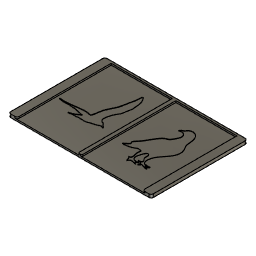
Wingspan - Lid alt (Autodesk Fusion 360 design; units mm, degrees)
Autodesk Fusion 360 part; units mm, degrees
sketch "Skizze1" plane through (0, 0, 0) normal (0, 0, 1) x (1, 0, 0)
  line L0 (0, 0) -> (135.5, 0)
  line L1 (135.5, 0) -> (135.5, 91.5)
  line L2 (135.5, 91.5) -> (0, 91.5)
  line L3 (0, 91.5) -> (0, 0)
  line L4 (0, 0) -> (7, 0)
  line L5 (7, 0) -> (7, 7)
  line L6 (7, 7) -> (0, 7)
  line L7 (0, 7) -> (0, 0)
  line L8 (135.5, 0) -> (128.5, 0)
  line L9 (128.5, 0) -> (128.5, 7)
  line L10 (128.5, 7) -> (135.5, 7)
  line L11 (135.5, 7) -> (135.5, 0)
  line L12 (135.5, 91.5) -> (128.5, 91.5)
  line L13 (128.5, 91.5) -> (128.5, 84.5)
  line L14 (128.5, 84.5) -> (135.5, 84.5)
  line L15 (135.5, 84.5) -> (135.5, 91.5)
  line L16 (0, 91.5) -> (7, 91.5)
  line L17 (7, 91.5) -> (7, 84.5)
  line L18 (7, 84.5) -> (0, 84.5)
  line L19 (0, 84.5) -> (0, 91.5)
  circle A0 centre (3.5, 88) radius 2.65
  circle A1 centre (132, 88) radius 2.65
  circle A2 centre (132, 3.5) radius 2.65
  circle A3 centre (3.5, 3.5) radius 2.65
  dimension "d1" = 135.5
  dimension "d2" = 91.5
  dimension "d3" = 7
  dimension "d4" = 7
  dimension "d5" = 7
  dimension "d6" = 7
  dimension "d7" = 7
  dimension "d8" = 7
  dimension "d9" = 7
  dimension "d10" = 7
  dimension "d11" = 5.3
  dimension "d12" = 5.3
  dimension "d13" = 5.3
  dimension "d14" = 5.3
  dimension "d15" = 3.5
  dimension "d16" = 3.5
  dimension "d17" = 3.5
  dimension "d18" = 3.5
  dimension "d19" = 3.5
  dimension "d20" = 3.5
  dimension "d21" = 3.5
  dimension "d22" = 3.5
  constraint horizontal L0
  constraint vertical L1
  constraint horizontal L2
  constraint vertical L3
  constraint coincident L0.start L3.end
  constraint horizontal L4
  constraint vertical L5
  constraint horizontal L6
  constraint vertical L7
  constraint horizontal L8
  constraint vertical L9
  constraint horizontal L10
  constraint vertical L11
  constraint horizontal L12
  constraint vertical L13
  constraint horizontal L14
  constraint vertical L15
  constraint horizontal L16
  constraint vertical L17
  constraint horizontal L18
  constraint vertical L19
  measures "d1" distance of L0.start L0.end
  measures "d2" distance of L0.start L2.end
  measures "d3" distance of L0.start L4.end
  measures "d4" distance of L0.start L6.end
  measures "d5" distance of L0.end L8.end
  measures "d6" distance of L0.end L10.end
  measures "d7" distance of L1.end L12.end
  measures "d8" distance of L1.end L14.end
  measures "d9" distance of L2.end L16.end
  measures "d10" distance of L2.end L18.end
  measures "d11" diameter of A0
  measures "d12" diameter of A1
  measures "d13" diameter of A2
  measures "d14" diameter of A3
  measures "d15" distance of L3 A3.centre
  measures "d16" distance of L6 A3.centre
  measures "d17" distance of L10 A2.centre
  measures "d18" distance of L1 A2.centre
  measures "d19" distance of L15 A1.centre
  measures "d20" distance of L12 A1.centre
  measures "d21" distance of L2 A0.centre
  measures "d22" distance of L17 A0.centre
extrude "Extrusion1" add sketch "Skizze1" along normal blind 3 contours L0 L3 L4 L5 L6 L7 | L0 L1 L2 L3 L5 L6 L9 L10 L13 L14 L17 L18 | L0 L1 L8 L9 L10 L11 | L2 L3 L16 L17 L18 L19 | L1 L2 L12 L13 L14 L15 | A0 | A1 | A2 | A3
extrude "Extrusion2" cut sketch "Skizze1" along normal blind 1.2 contours A0 | A1 | A2 | A3
sketch "Skizze2" plane through (0, 0, 3) normal (0, 0, 1) x (-1, 0, 0)
  line L0 (0, -91.5) -> (0, 0)
  line L1 (0, 0) -> (-135.5, 0)
  line L2 (-135.5, 0) -> (-135.5, -91.5)
  line L3 (-135.5, -91.5) -> (0, -91.5)
  line L4 (-8, 0) -> (-66, 0)
  line L5 (-66, 0) -> (-66, -89.5)
  line L6 (-66, -89.5) -> (-8, -89.5)
  line L7 (-8, -89.5) -> (-8, 0)
  line L8 (-69.5, 0) -> (-127.5, 0)
  line L9 (-127.5, 0) -> (-127.5, -89.5)
  line L10 (-127.5, -89.5) -> (-69.5, -89.5)
  line L11 (-69.5, -89.5) -> (-69.5, 0)
  dimension "d27" = 2
  dimension "d28" = 2
  dimension "d29" = 58
  dimension "d30" = 58
  dimension "d31" = 8
  dimension "d32" = 8
  constraint horizontal L4
  constraint vertical L5
  constraint horizontal L6
  constraint vertical L7
  constraint coincident L1 L4.start
  constraint horizontal L8
  constraint vertical L9
  constraint horizontal L10
  constraint vertical L11
  constraint coincident L1 L8.start
  measures "d27" distance of L3 L6
  measures "d28" distance of L3 L10
  measures "d29" distance of L5 L7
  measures "d30" distance of L9 L11
  measures "d31" distance of L0 L7
  measures "d32" distance of L2 L9
extrude "Extrusion3" cut sketch "Skizze2" against normal blind 1.5 contours L1 L4 L5 L6 L7 | L1 L8 L9 L10 L11
sketch "Skizze3" plane through (0, 0, 1.5) normal (0, 0, 1) x (-1, 0, 0)
  line L0 (-8, -89.5) -> (-8, 0)
  line L1 (-8, 0) -> (-66, 0)
  line L2 (-66, 0) -> (-66, -89.5)
  line L3 (-66, -89.5) -> (-8, -89.5)
  spline S0 degree 3 poles (-54.6107, -35.5203) (-54.3857, -35.6587) (-54.1474, -35.7829) (-53.9016, -35.8782) knots 0 0 0 0 1 1 1 1
  spline S1 degree 3 poles (-53.9016, -35.8782) (-53.3812, -36.0798) (-53.0237, -36.4468) (-52.8933, -36.9716) knots 0 0 0 0 1 1 1 1
  spline S2 degree 3 poles (-52.8933, -36.9716) (-52.7024, -37.7411) (-52.1061, -38.0808) (-51.4599, -38.1653) knots 0 0 0 0 1 1 1 1
  spline S3 degree 3 poles (-51.4599, -38.1653) (-50.2172, -38.3273) (-49.4416, -39.1533) (-48.7794, -40.0184) knots 0 0 0 0 1 1 1 1
  spline S4 degree 3 poles (-48.7794, -40.0184) (-48.2854, -40.664) (-48.0987, -41.5504) (-48.405, -42.4175) knots 0 0 0 0 1 1 1 1
  spline S5 degree 3 poles (-48.405, -42.4175) (-48.4756, -42.6178) (-48.4813, -42.7792) (-48.4006, -43.0131) knots 0 0 0 0 1 1 1 1
  spline S6 degree 3 poles (-48.4006, -43.0131) (-48.2992, -43.3059) (-48.4121, -43.6773) (-48.4492, -44.013) knots 0 0 0 0 1 1 1 1
  spline S7 degree 3 poles (-48.4492, -44.013) (-48.8132, -47.3059) (-50.1119, -50.2491) (-51.8343, -53.0328) knots 0 0 0 0 1 1 1 1
  spline S8 degree 3 poles (-51.8343, -53.0328) (-51.9971, -53.2959) (-52.1599, -53.5586) (-52.3243, -53.8203) knots 0 0 0 0 1 1 1 1
  spline S9 degree 3 poles (-52.3243, -53.8203) (-52.7467, -54.4933) (-52.9206, -55.2199) (-53.0199, -56.0179) knots 0 0 0 0 1 1 1 1
  spline S10 degree 3 poles (-53.0199, -56.0179) (-53.2299, -57.7055) (-53.2931, -59.4168) (-53.807, -61.0654) knots 0 0 0 0 1 1 1 1
  spline S11 degree 3 poles (-53.807, -61.0654) (-54.3381, -62.7692) (-54.2997, -64.5059) (-53.989, -66.2604) knots 0 0 0 0 1 1 1 1
  spline S12 degree 3 poles (-53.989, -66.2604) (-53.8286, -67.1668) (-53.8651, -68.1065) (-53.7711, -69.027) knots 0 0 0 0 1 1 1 1
  spline S13 degree 3 poles (-53.7711, -69.027) (-53.5564, -71.1385) (-53.063, -73.1793) (-52.0325, -75.052) knots 0 0 0 0 1 1 1 1
  spline S14 degree 3 poles (-52.0325, -75.052) (-51.5732, -75.8865) (-51.0371, -76.6799) (-50.5086, -77.4742) knots 0 0 0 0 1 1 1 1
  spline S15 degree 3 poles (-50.5086, -77.4742) (-50.2908, -77.8014) (-50.0332, -78.1471) (-49.5381, -77.9648) knots 0 0 0 0 1 1 1 1
  spline S16 degree 3 poles (-49.5381, -77.9648) (-49.2777, -77.8689) (-48.9313, -77.2061) (-48.9526, -76.8461) knots 0 0 0 0 1 1 1 1
  spline S17 degree 3 poles (-48.9526, -76.8461) (-48.9587, -76.7441) (-49.0093, -76.6408) (-48.9986, -76.5426) knots 0 0 0 0 1 1 1 1
  spline S18 degree 3 poles (-48.9986, -76.5426) (-48.976, -76.3359) (-48.927, -76.1323) (-48.8877, -75.9273) knots 0 0 0 0 1 1 1 1
  spline S19 degree 3 poles (-48.8877, -75.9273) (-48.8294, -75.6205) (-48.7527, -75.3155) (-48.7166, -75.0062) knots 0 0 0 0 1 1 1 1
  spline S20 degree 3 poles (-48.7166, -75.0062) (-48.6832, -74.7202) (-48.6916, -74.4288) (-48.6841, -74.1398) knots 0 0 0 0 1 1 1 1
  spline S21 degree 3 poles (-48.6841, -74.1398) (-48.6757, -73.8024) (-48.6511, -73.4641) (-48.6683, -73.1281) knots 0 0 0 0 1 1 1 1
  spline S22 degree 3 poles (-48.6683, -73.1281) (-48.6967, -72.5702) (-48.7331, -72.0357) (-48.4542, -71.4978) knots 0 0 0 0 1 1 1 1
  spline S23 degree 3 poles (-48.4542, -71.4978) (-48.3037, -71.2071) (-48.388, -70.8025) (-48.3205, -70.4585) knots 0 0 0 0 1 1 1 1
  spline S24 degree 3 poles (-48.3205, -70.4585) (-48.2493, -70.0955) (-48.1155, -69.7453) (-48.0227, -69.3864) knots 0 0 0 0 1 1 1 1
  spline S25 degree 3 poles (-48.0227, -69.3864) (-47.8829, -68.8474) (-47.7289, -68.3102) (-47.6279, -67.7636) knots 0 0 0 0 1 1 1 1
  spline S26 degree 3 poles (-47.6279, -67.7636) (-47.4516, -66.8124) (-47.3396, -65.8486) (-47.1484, -64.9005) knots 0 0 0 0 1 1 1 1
  spline S27 degree 3 poles (-47.1484, -64.9005) (-46.8988, -63.6623) (-46.5909, -62.4358) (-46.3234, -61.2009) knots 0 0 0 0 1 1 1 1
  spline S28 degree 3 poles (-46.3234, -61.2009) (-46.209, -60.6725) (-46.1431, -60.1335) (-46.0354, -59.6034) knots 0 0 0 0 1 1 1 1
  spline S29 degree 3 poles (-46.0354, -59.6034) (-45.9983, -59.4207) (-45.894, -59.2526) (-45.8332, -59.0736) knots 0 0 0 0 1 1 1 1
  spline S30 degree 3 poles (-45.8332, -59.0736) (-45.7289, -58.7653) (-45.6329, -58.4544) (-45.5384, -58.143) knots 0 0 0 0 1 1 1 1
  spline S31 degree 3 poles (-45.5384, -58.143) (-45.5219, -58.0883) (-45.5458, -58.0181) (-45.5225, -57.9685) knots 0 0 0 0 1 1 1 1
  spline S32 degree 3 poles (-45.5225, -57.9685) (-45.2163, -57.3208) (-44.9036, -56.6766) (-44.5954, -56.0299) knots 0 0 0 0 1 1 1 1
  spline S33 degree 3 poles (-44.5954, -56.0299) (-44.4278, -55.6788) (-44.2644, -55.3252) (-44.1023, -54.9717) knots 0 0 0 0 1 1 1 1
  spline S34 degree 3 poles (-44.1023, -54.9717) (-44.072, -54.9054) (-44.0628, -54.8295) (-44.0317, -54.7636) knots 0 0 0 0 1 1 1 1
  spline S35 degree 3 poles (-44.0317, -54.7636) (-43.3787, -53.3887) (-42.6824, -52.0319) (-42.0803, -50.6349) knots 0 0 0 0 1 1 1 1
  spline S36 degree 3 poles (-42.0803, -50.6349) (-41.4158, -49.093) (-40.9656, -47.4902) (-40.7678, -45.8035) knots 0 0 0 0 1 1 1 1
  spline S37 degree 3 poles (-40.7678, -45.8035) (-40.5659, -44.0848) (-40.2289, -42.3806) (-39.9081, -40.6779) knots 0 0 0 0 1 1 1 1
  spline S38 degree 3 poles (-39.9081, -40.6779) (-39.8095, -40.1549) (-39.5825, -39.6535) (-39.3888, -39.1524) knots 0 0 0 0 1 1 1 1
  spline S39 degree 3 poles (-39.3888, -39.1524) (-39.2638, -38.8288) (-38.8053, -38.6563) (-38.4481, -38.7397) knots 0 0 0 0 1 1 1 1
  spline S40 degree 3 poles (-38.4481, -38.7397) (-36.5558, -39.1814) (-34.657, -39.6589) (-32.706, -39.6251) knots 0 0 0 0 1 1 1 1
  spline S41 degree 3 poles (-32.706, -39.6251) (-31.5376, -39.6048) (-30.3757, -39.3138) (-29.2077, -39.1685) knots 0 0 0 0 1 1 1 1
  spline S42 degree 3 poles (-29.2077, -39.1685) (-25.6736, -38.7295) (-22.1402, -38.2858) (-18.6027, -37.8763) knots 0 0 0 0 1 1 1 1
  spline S43 degree 3 poles (-18.6027, -37.8763) (-16.1104, -37.5876) (-13.613, -37.5339) (-11.1203, -37.9066) knots 0 0 0 0 1 1 1 1
  spline S44 degree 3 poles (-11.1203, -37.9066) (-10.9896, -37.9262) (-10.8569, -37.9337) (-10.7245, -37.9374) knots 0 0 0 0 1 1 1 1
  spline S45 degree 3 poles (-10.7245, -37.9374) (-10.6864, -37.9384) (-10.6472, -37.9074) (-10.5118, -37.8495) knots 0 0 0 0 1 1 1 1
  spline S46 degree 3 poles (-10.5118, -37.8495) (-10.7016, -37.7155) (-10.8174, -37.5784) (-10.9589, -37.5426) knots 0 0 0 0 1 1 1 1
  spline S47 degree 3 poles (-10.9589, -37.5426) (-11.5843, -37.3856) (-12.2151, -37.2472) (-12.8479, -37.1222) knots 0 0 0 0 1 1 1 1
  spline S48 degree 3 poles (-12.8479, -37.1222) (-13.3776, -37.0175) (-13.9244, -36.9827) (-14.444, -36.8433) knots 0 0 0 0 1 1 1 1
  spline S49 degree 3 poles (-14.444, -36.8433) (-15.64, -36.5218) (-16.8287, -36.6495) (-18.029, -36.7886) knots 0 0 0 0 1 1 1 1
  spline S50 degree 3 poles (-18.029, -36.7886) (-19.0309, -36.9047) (-20.0388, -36.997) (-21.0461, -37.0236) knots 0 0 0 0 1 1 1 1
  spline S51 degree 3 poles (-21.0461, -37.0236) (-21.4277, -37.0337) (-21.8093, -36.7946) (-22.2007, -36.7346) knots 0 0 0 0 1 1 1 1
  spline S52 degree 3 poles (-22.2007, -36.7346) (-22.6265, -36.6691) (-23.0637, -36.6702) (-23.4963, -36.659) knots 0 0 0 0 1 1 1 1
  spline S53 degree 3 poles (-23.4963, -36.659) (-23.9903, -36.6462) (-24.485, -36.6549) (-24.979, -36.6492) knots 0 0 0 0 1 1 1 1
  spline S54 degree 3 poles (-24.979, -36.6492) (-25.5074, -36.6428) (-26.0467, -36.6955) (-26.5613, -36.606) knots 0 0 0 0 1 1 1 1
  spline S55 degree 3 poles (-26.5613, -36.606) (-27.3947, -36.4608) (-28.2125, -36.2231) (-29.0354, -36.0198) knots 0 0 0 0 1 1 1 1
  spline S56 degree 3 poles (-29.0354, -36.0198) (-29.8563, -35.8169) (-30.6749, -35.6035) (-31.4967, -35.4032) knots 0 0 0 0 1 1 1 1
  spline S57 degree 3 poles (-31.4967, -35.4032) (-32.0765, -35.2618) (-32.6596, -35.1325) (-33.2425, -35.0045) knots 0 0 0 0 1 1 1 1
  spline S58 degree 3 poles (-33.2425, -35.0045) (-33.3252, -34.9863) (-33.4319, -34.9744) (-33.5008, -35.0105) knots 0 0 0 0 1 1 1 1
  spline S59 degree 3 poles (-33.5008, -35.0105) (-33.8193, -35.1784) (-33.9951, -35.0615) (-34.0674, -34.6911) knots 0 0 0 0 1 1 1 1
  spline S60 degree 3 poles (-34.0674, -34.6911) (-34.4368, -34.803) (-34.7701, -34.9038) (-35.1037, -35.0048) knots 0 0 0 0 1 1 1 1
  spline S61 degree 3 poles (-35.1037, -35.0048) (-35.1294, -34.966) (-35.1554, -34.9272) (-35.181, -34.8884) knots 0 0 0 0 1 1 1 1
  spline S62 degree 3 poles (-35.181, -34.8884) (-33.7672, -33.9398) (-32.3787, -32.9505) (-30.9325, -32.0543) knots 0 0 0 0 1 1 1 1
  spline S63 degree 3 poles (-30.9325, -32.0543) (-29.4765, -31.1524) (-27.8141, -30.7573) (-26.1326, -30.4433) knots 0 0 0 0 1 1 1 1
  spline S64 degree 3 poles (-26.1326, -30.4433) (-26.1403, -30.373) (-26.1481, -30.3028) (-26.1559, -30.2322) knots 0 0 0 0 1 1 1 1
  spline S65 degree 3 poles (-26.1559, -30.2322) (-26.5311, -30.1761) (-26.9228, -30.0222) (-27.2777, -30.0833) knots 0 0 0 0 1 1 1 1
  spline S66 degree 3 poles (-27.2777, -30.0833) (-28.1481, -30.2332) (-29.0011, -30.4837) (-29.8618, -30.6907) knots 0 0 0 0 1 1 1 1
  spline S67 degree 3 poles (-29.8618, -30.6907) (-30.0337, -30.732) (-30.1779, -30.8151) (-30.3511, -30.5952) knots 0 0 0 0 1 1 1 1
  spline S68 degree 3 poles (-30.3511, -30.5952) (-30.4446, -30.4763) (-30.7634, -30.4986) (-30.9758, -30.5165) knots 0 0 0 0 1 1 1 1
  spline S69 degree 3 poles (-30.9758, -30.5165) (-31.5029, -30.5611) (-32.0256, -30.6597) (-32.5527, -30.6973) knots 0 0 0 0 1 1 1 1
  spline S70 degree 3 poles (-32.5527, -30.6973) (-32.884, -30.7209) (-33.2206, -30.6729) (-33.5548, -30.659) knots 0 0 0 0 1 1 1 1
  spline S71 degree 3 poles (-33.5548, -30.659) (-33.6852, -30.6537) (-33.8472, -30.602) (-33.9418, -30.659) knots 0 0 0 0 1 1 1 1
  spline S72 degree 3 poles (-33.9418, -30.659) (-34.7269, -31.1355) (-35.6016, -30.9569) (-36.4305, -30.968) knots 0 0 0 0 1 1 1 1
  spline S73 degree 3 poles (-36.4305, -30.968) (-37.766, -30.986) (-39.1058, -30.911) (-40.4394, -30.8154) knots 0 0 0 0 1 1 1 1
  spline S74 degree 3 poles (-40.4394, -30.8154) (-41.7411, -30.7222) (-42.9698, -30.9535) (-44.156, -31.4641) knots 0 0 0 0 1 1 1 1
  spline S75 degree 3 poles (-44.156, -31.4641) (-45.7394, -32.1458) (-47.3565, -32.7091) (-49.0432, -33.095) knots 0 0 0 0 1 1 1 1
  spline S76 degree 3 poles (-49.0432, -33.095) (-49.9886, -33.3114) (-50.9395, -33.5471) (-51.7567, -34.1779) knots 0 0 0 0 1 1 1 1
  spline S77 degree 3 poles (-51.7567, -34.1779) (-52.4884, -34.7425) (-53.3623, -34.7554) (-54.2355, -34.4366) knots 0 0 0 0 1 1 1 1
  spline S78 degree 3 poles (-54.2355, -34.4366) (-54.6698, -34.2778) (-55.1162, -34.1522) (-55.6479, -33.9828) knots 0 0 0 0 1 1 1 1
  spline S79 degree 3 poles (-55.6479, -33.9828) (-55.5045, -34.7139) (-55.1551, -35.186) (-54.6107, -35.5203) knots 0 0 0 0 1 1 1 1
extrude "Extrusion4" cut sketch "Skizze3" against normal blind 0.4 contours S0 S1 S2 S3 S4 S5 S6 S7 S8 S9 S10 S11 S12 S13 S14 S15 S16 S17 S18 S19 S20 S21 S22 S23 S24 S25 S26 S27 S28 S29 S30 S31 S32 S33 S34 S35 S36 S37 S38 S39 S40 S41 S42 S43 S44 S45 S46 S47 S48 S49 S50 S51 S52 S53 S54 S55 S56 S57 S58 S59 S60 S61 S62 S63 S64 S65 S66 S67 S68 S69 S70 S71 S72 S73 S74 S75 S76 S77 S78 S79
sketch "Skizze4" plane through (0, 0, 1.5) normal (0, 0, 1) x (-1, 0, 0)
  line L0 (-69.5, -89.5) -> (-69.5, 0)
  line L1 (-69.5, 0) -> (-127.5, 0)
  line L2 (-127.5, 0) -> (-127.5, -89.5)
  line L3 (-127.5, -89.5) -> (-69.5, -89.5)
  spline S0 degree 3 poles (-109.5849, -59.8174) (-109.2406, -61.5753) (-109.2707, -63.4131) (-108.9799, -65.1849) knots 0 0 0 0 1 1 1 1
  spline S1 degree 3 poles (-108.9799, -65.1849) (-108.5845, -67.5934) (-107.7601, -70.0419) (-106.0022, -71.7349) knots 0 0 0 0 1 1 1 1
  spline S2 degree 3 poles (-106.0022, -71.7349) (-103.8217, -73.8351) (-100.5666, -74.0342) (-98.1392, -72.2525) knots 0 0 0 0 1 1 1 1
  spline S3 degree 3 poles (-98.1392, -72.2525) (-97.9155, -72.0887) (-97.8519, -71.6996) (-97.7299, -71.4072) knots 0 0 0 0 1 1 1 1
  spline S4 degree 3 poles (-97.7299, -71.4072) (-97.6915, -71.3149) (-97.6598, -71.2196) (-97.6278, -71.117) knots 0 0 0 0 1 1 1 1
  spline S5 degree 3 poles (-97.6278, -71.117) (-97.5772, -70.9548) (-97.4928, -70.7866) (-97.4386, -70.7427) knots 0 0 0 0 1 1 1 1
  spline S6 degree 3 poles (-97.4386, -70.7427) (-97.4058, -70.7162) (-97.3734, -70.6897) (-97.3405, -70.6632) knots 0 0 0 0 1 1 1 1
  spline S7 degree 3 poles (-97.3405, -70.6632) (-97.3215, -70.6478) (-97.3041, -70.6308) (-97.2874, -70.6126) knots 0 0 0 0 1 1 1 1
  spline S8 degree 3 poles (-97.2874, -70.6126) (-97.2606, -70.5829) (-97.0879, -70.4685) (-96.896, -70.3637) knots 0 0 0 0 1 1 1 1
  spline S9 degree 3 poles (-96.896, -70.3637) (-96.2284, -69.9988) (-95.5537, -69.6588) (-94.9715, -69.2013) knots 0 0 0 0 1 1 1 1
  spline S10 degree 3 poles (-94.9715, -69.2013) (-94.6035, -68.9121) (-94.3581, -68.4664) (-94.0954, -68.043) knots 0 0 0 0 1 1 1 1
  spline S11 degree 3 poles (-94.0954, -68.043) (-93.9798, -67.8573) (-93.9121, -67.6805) (-93.9536, -67.6413) knots 0 0 0 0 1 1 1 1
  spline S12 degree 3 poles (-93.9536, -67.6413) (-93.9953, -67.6022) (-94.2038, -67.5998) (-94.4199, -67.6343) knots 0 0 0 0 1 1 1 1
  spline S13 degree 3 poles (-94.4199, -67.6343) (-94.5786, -67.6596) (-94.7341, -67.6912) (-94.8754, -67.7554) knots 0 0 0 0 1 1 1 1
  spline S14 degree 3 poles (-94.8754, -67.7554) (-97.4827, -68.9367) (-100.315, -67.1831) (-100.4654, -64.3254) knots 0 0 0 0 1 1 1 1
  spline S15 degree 3 poles (-100.4654, -64.3254) (-100.5557, -62.6126) (-99.795, -60.9735) (-98.9276, -59.4941) knots 0 0 0 0 1 1 1 1
  spline S16 degree 3 poles (-98.9276, -59.4941) (-98.2959, -58.4172) (-97.4646, -56.6371) (-96.4463, -55.8868) knots 0 0 0 0 1 1 1 1
  spline S17 degree 3 poles (-96.4463, -55.8868) (-95.5704, -55.2414) (-94.619, -55.3083) (-93.6664, -54.7222) knots 0 0 0 0 1 1 1 1
  spline S18 degree 3 poles (-93.6664, -54.7222) (-91.5073, -53.394) (-89.9733, -50.5573) (-88.7053, -48.4559) knots 0 0 0 0 1 1 1 1
  spline S19 degree 3 poles (-88.7053, -48.4559) (-87.4646, -46.4) (-86.3657, -44.261) (-85.0747, -42.2371) knots 0 0 0 0 1 1 1 1
  spline S20 degree 3 poles (-85.0747, -42.2371) (-83.8673, -40.3438) (-82.2285, -38.8242) (-80.9178, -37.0916) knots 0 0 0 0 1 1 1 1
  spline S21 degree 3 poles (-80.9178, -37.0916) (-80.7861, -36.9175) (-80.7599, -36.6171) (-80.8284, -36.4097) knots 0 0 0 0 1 1 1 1
  spline S22 degree 3 poles (-80.8284, -36.4097) (-80.8866, -36.2344) (-80.9498, -36.0232) (-80.9938, -35.8407) knots 0 0 0 0 1 1 1 1
  spline S23 degree 3 poles (-80.9938, -35.8407) (-81.0453, -35.6282) (-81.2328, -35.435) (-81.4141, -35.3132) knots 0 0 0 0 1 1 1 1
  spline S24 degree 3 poles (-81.4141, -35.3132) (-82.5178, -34.5704) (-78.814, -31.7234) (-77.6521, -30.7657) knots 0 0 0 0 1 1 1 1
  spline S25 degree 3 poles (-77.6521, -30.7657) (-77.4835, -30.6267) (-77.529, -30.4807) (-77.7463, -30.4582) knots 0 0 0 0 1 1 1 1
  spline S26 degree 3 poles (-77.7463, -30.4582) (-80.6963, -30.153) (-83.9624, -31.0747) (-86.566, -32.1207) knots 0 0 0 0 1 1 1 1
  spline S27 degree 3 poles (-86.566, -32.1207) (-86.835, -32.2288) (-87.0852, -32.3906) (-87.3314, -32.5473) knots 0 0 0 0 1 1 1 1
  spline S28 degree 3 poles (-87.3314, -32.5473) (-87.7745, -32.8295) (-88.2032, -33.1346) (-88.6464, -33.4168) knots 0 0 0 0 1 1 1 1
  spline S29 degree 3 poles (-88.6464, -33.4168) (-89.119, -33.7176) (-93.2561, -33.7452) (-92.7999, -32.8402) knots 0 0 0 0 1 1 1 1
  spline S30 degree 3 poles (-92.7999, -32.8402) (-91.6558, -30.5714) (-92.868, -28.2245) (-93.2474, -25.9411) knots 0 0 0 0 1 1 1 1
  spline S31 degree 3 poles (-93.2474, -25.9411) (-93.4021, -25.0115) (-93.2482, -24.2667) (-93.0828, -23.5353) knots 0 0 0 0 1 1 1 1
  spline S32 degree 3 poles (-93.0828, -23.5353) (-93.0345, -23.322) (-92.8208, -23.1233) (-92.6059, -23.0838) knots 0 0 0 0 1 1 1 1
  spline S33 degree 3 poles (-92.6059, -23.0838) (-91.8092, -22.9369) (-91.0883, -22.7106) (-91.6486, -22.4138) knots 0 0 0 0 1 1 1 1
  spline S34 degree 3 poles (-91.6486, -22.4138) (-92.0851, -22.1827) (-92.3934, -21.8986) (-92.6047, -21.6453) knots 0 0 0 0 1 1 1 1
  spline S35 degree 3 poles (-92.6047, -21.6453) (-92.7448, -21.4775) (-92.8524, -21.1486) (-92.8889, -20.9329) knots 0 0 0 0 1 1 1 1
  spline S36 degree 3 poles (-92.8889, -20.9329) (-93.0234, -20.1291) (-93.3238, -19.3021) (-93.5945, -18.5525) knots 0 0 0 0 1 1 1 1
  spline S37 degree 3 poles (-93.5945, -18.5525) (-93.6689, -18.3471) (-93.8232, -18.3297) (-93.9356, -18.5173) knots 0 0 0 0 1 1 1 1
  spline S38 degree 3 poles (-93.9356, -18.5173) (-94.8795, -20.0904) (-95.124, -20.9994) (-97.0391, -20.5704) knots 0 0 0 0 1 1 1 1
  spline S39 degree 3 poles (-97.0391, -20.5704) (-98.3004, -20.2882) (-99.585, -19.9052) (-100.8483, -19.6373) knots 0 0 0 0 1 1 1 1
  spline S40 degree 3 poles (-100.8483, -19.6373) (-101.0624, -19.5917) (-101.0921, -19.6622) (-100.9151, -19.7908) knots 0 0 0 0 1 1 1 1
  spline S41 degree 3 poles (-100.9151, -19.7908) (-100.2831, -20.2507) (-99.6543, -20.7184) (-98.991, -21.1311) knots 0 0 0 0 1 1 1 1
  spline S42 degree 3 poles (-98.991, -21.1311) (-98.8053, -21.2467) (-98.8208, -21.2772) (-99.0369, -21.2464) knots 0 0 0 0 1 1 1 1
  spline S43 degree 3 poles (-99.0369, -21.2464) (-100.1754, -21.0837) (-100.468, -22.0355) (-101.1328, -22.4245) knots 0 0 0 0 1 1 1 1
  spline S44 degree 3 poles (-101.1328, -22.4245) (-101.3216, -22.535) (-101.3267, -22.531) (-101.1117, -22.491) knots 0 0 0 0 1 1 1 1
  spline S45 degree 3 poles (-101.1117, -22.491) (-100.1576, -22.3145) (-99.1916, -22.1665) (-98.2283, -22.2603) knots 0 0 0 0 1 1 1 1
  spline S46 degree 3 poles (-98.2283, -22.2603) (-95.3845, -22.5369) (-94.5367, -24.856) (-95.003, -27.5273) knots 0 0 0 0 1 1 1 1
  spline S47 degree 3 poles (-95.003, -27.5273) (-95.2459, -28.9203) (-96.51, -33.5265) (-97.9525, -34.0801) knots 0 0 0 0 1 1 1 1
  spline S48 degree 3 poles (-97.9525, -34.0801) (-98.6672, -34.3544) (-99.4857, -33.8214) (-99.8027, -33.1247) knots 0 0 0 0 1 1 1 1
  spline S49 degree 3 poles (-99.8027, -33.1247) (-100.12, -32.4286) (-100.0702, -31.6281) (-100.0207, -30.8646) knots 0 0 0 0 1 1 1 1
  spline S50 degree 3 poles (-100.0207, -30.8646) (-99.9712, -30.1012) (-99.9356, -29.2971) (-100.2755, -28.6115) knots 0 0 0 0 1 1 1 1
  spline S51 degree 3 poles (-100.2755, -28.6115) (-100.5807, -27.9966) (-101.1466, -27.5616) (-101.6092, -27.0543) knots 0 0 0 0 1 1 1 1
  spline S52 degree 3 poles (-101.6092, -27.0543) (-102.0719, -26.5473) (-102.4557, -25.858) (-102.267, -25.1982) knots 0 0 0 0 1 1 1 1
  spline S53 degree 3 poles (-102.267, -25.1982) (-102.0975, -24.605) (-101.4968, -24.2172) (-100.8889, -24.113) knots 0 0 0 0 1 1 1 1
  spline S54 degree 3 poles (-100.8889, -24.113) (-100.4105, -24.031) (-99.9237, -24.0921) (-99.4437, -24.1831) knots 0 0 0 0 1 1 1 1
  spline S55 degree 3 poles (-99.4437, -24.1831) (-99.2288, -24.2239) (-99.1489, -24.1055) (-99.3166, -23.9655) knots 0 0 0 0 1 1 1 1
  spline S56 degree 3 poles (-99.3166, -23.9655) (-100.4881, -22.9872) (-103.322, -23.9124) (-102.7257, -21.7979) knots 0 0 0 0 1 1 1 1
  spline S57 degree 3 poles (-102.7257, -21.7979) (-102.6022, -21.361) (-102.5029, -20.917) (-102.3972, -20.4618) knots 0 0 0 0 1 1 1 1
  spline S58 degree 3 poles (-102.3972, -20.4618) (-102.3477, -20.249) (-102.4684, -20.15) (-102.6588, -20.2574) knots 0 0 0 0 1 1 1 1
  spline S59 degree 3 poles (-102.6588, -20.2574) (-103.4577, -20.7061) (-103.9659, -21.3128) (-103.8416, -22.3374) knots 0 0 0 0 1 1 1 1
  spline S60 degree 3 poles (-103.8416, -22.3374) (-103.8266, -22.462) (-108.4552, -21.0792) (-108.7533, -20.9831) knots 0 0 0 0 1 1 1 1
  spline S61 degree 3 poles (-108.7533, -20.9831) (-109.1122, -20.8672) (-109.4906, -20.8094) (-109.9097, -20.7362) knots 0 0 0 0 1 1 1 1
  spline S62 degree 3 poles (-109.9097, -20.7362) (-110.1249, -20.6985) (-110.248, -20.8339) (-110.1724, -21.0389) knots 0 0 0 0 1 1 1 1
  spline S63 degree 3 poles (-110.1724, -21.0389) (-109.9556, -21.6289) (-109.6853, -22.0294) (-109.0085, -22.1497) knots 0 0 0 0 1 1 1 1
  spline S64 degree 3 poles (-109.0085, -22.1497) (-108.3627, -22.2649) (-107.72, -22.4584) (-107.0983, -22.6788) knots 0 0 0 0 1 1 1 1
  spline S65 degree 3 poles (-107.0983, -22.6788) (-106.8921, -22.7517) (-106.9032, -22.8178) (-107.1216, -22.8067) knots 0 0 0 0 1 1 1 1
  spline S66 degree 3 poles (-107.1216, -22.8067) (-108.2871, -22.7488) (-110.7142, -22.4777) (-110.7189, -23.6789) knots 0 0 0 0 1 1 1 1
  spline S67 degree 3 poles (-110.7189, -23.6789) (-110.7198, -23.8973) (-110.4756, -24.0377) (-110.2615, -23.9943) knots 0 0 0 0 1 1 1 1
  spline S68 degree 3 poles (-110.2615, -23.9943) (-109.8495, -23.91) (-109.4351, -23.8139) (-109.0227, -23.8229) knots 0 0 0 0 1 1 1 1
  spline S69 degree 3 poles (-109.0227, -23.8229) (-107.4722, -23.8576) (-105.7114, -23.5834) (-104.5409, -24.61) knots 0 0 0 0 1 1 1 1
  spline S70 degree 3 poles (-104.5409, -24.61) (-103.3928, -25.6164) (-103.1324, -27.8318) (-103.2278, -29.2402) knots 0 0 0 0 1 1 1 1
  spline S71 degree 3 poles (-103.2278, -29.2402) (-103.713, -36.4175) (-110.9191, -40.3251) (-112.9933, -47.0184) knots 0 0 0 0 1 1 1 1
  spline S72 degree 3 poles (-112.9933, -47.0184) (-113.9953, -50.2529) (-113.1813, -53.1537) (-111.4962, -55.9777) knots 0 0 0 0 1 1 1 1
  spline S73 degree 3 poles (-111.4962, -55.9777) (-110.6463, -57.4033) (-109.9046, -58.1849) (-109.5849, -59.8174) knots 0 0 0 0 1 1 1 1
extrude "Extrusion5" cut sketch "Skizze4" against normal blind 0.4 contours S0 S1 S2 S3 S4 S5 S6 S7 S8 S9 S10 S11 S12 S13 S14 S15 S16 S17 S18 S19 S20 S21 S22 S23 S24 S25 S26 S27 S28 S29 S30 S31 S32 S33 S34 S35 S36 S37 S38 S39 S40 S41 S42 S43 S44 S45 S46 S47 S48 S49 S50 S51 S52 S53 S54 S55 S56 S57 S58 S59 S60 S61 S62 S63 S64 S65 S66 S67 S68 S69 S70 S71 S72 S73
fillet "Abrundung1" radius 2 4 edges at (8, 0, 2.25) (0, 0, 1.5) (135.5, 0, 1.5) (127.5, 0, 2.25)
fillet "Abrundung2" radius 2 2 edges at (135.5, 91.5, 1.5) (0, 91.5, 1.5)
fillet "Abrundung3" radius 1 2 edges at (66, 0, 2.25) (69.5, 0, 2.25)
